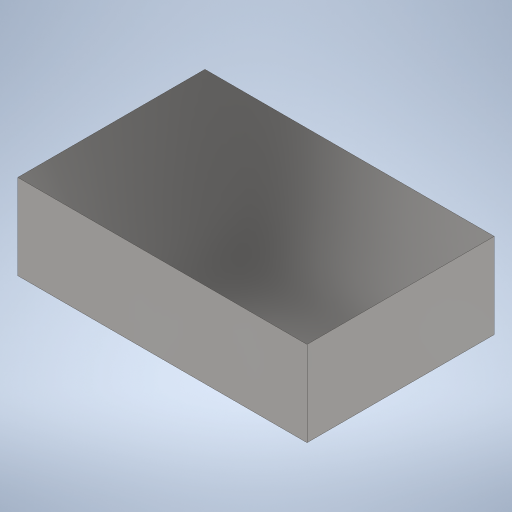
# Autodesk Inventor part: Circuit
Saved by Autodesk Inventor 2023 (Build 270158000, 158)
## iProperties
Created: 2023-04-05
Part Number: Circuit
Material: Generic
Document SubType Name: Modeling
Designer: IanJm
Density: 1 g/cm^3
Appearance: Galvanized
Author: IanJm
Autodesk Inventor part; units mm, degrees
ref_plane "YZ Plane" through (0, 0, 0) normal (1, 0, 0) x (0, 1, 0)
ref_plane "XZ Plane" through (0, 0, 0) normal (0, 1, 0) x (-1, 0, 0)
ref_plane "XY Plane" through (0, 0, 0) normal (0, 0, 1) x (1, 0, 0)
sketch "Sketch1" plane through (0, 0, 0) normal (0, 1, 0) x (-1, 0, 0)
  line L0 (0, 0) -> (0, -55)
  line L1 (0, -55) -> (85, -55)
  line L2 (85, -55) -> (85, 0)
  line L3 (85, 0) -> (0, 0)
  dimension "d0" = 55
  dimension "d1" = 85
  constraints: 8 end point, 2 vertical, 1 horizontal, 1 perpendicular
  measures "d0" distance of L0.start L0.end
  measures "d1" distance of L0.end L1.end
extrude "Extrusion1" add sketch "Sketch1" along normal blind 25
body "Solid1"
